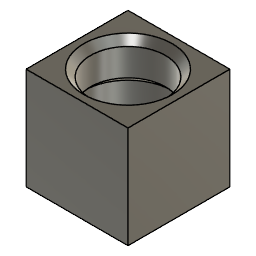
Peg hole_v1 (Autodesk Fusion 360 design; units mm, degrees)
part number: 2026-01-19-15-04-58-543
Autodesk Fusion 360 part; units mm, degrees
sketch "Sketch1" plane through (0, 0, 0) normal (0, 0, 1) x (1, 0, 0)
  line L0 (-19.05, -19.05) -> (19.05, -19.05)
  line L1 (19.05, -19.05) -> (19.05, 19.05)
  line L2 (19.05, 19.05) -> (-19.05, 19.05)
  line L3 (-19.05, 19.05) -> (-19.05, -19.05)
  line L4 (0, 1.75) -> (0, 22.5)
  line L5 (1.75, 0) -> (22.5, 0)
  dimension "d1" = 38.1
  dimension "d2" = 38.1
  constraint horizontal L0
  constraint vertical L1
  constraint horizontal L2
  constraint vertical L3
  constraint symmetric L1 L3 L4
  constraint symmetric L0 L2 L5
  measures "d1" distance of L1 L3
  measures "d2" distance of L0 L2
extrude "Extrude1" add sketch "Sketch1" along normal blind 38.1
sketch "Sketch2" plane through (0, 0, 38.1) normal (0, 0, 1) x (-1, 0, 0)
  line L0 (19.05, -19.05) -> (19.05, 19.05)
  line L1 (19.05, 19.05) -> (-19.05, 19.05)
  line L2 (-19.05, 19.05) -> (-19.05, -19.05)
  line L3 (-19.05, -19.05) -> (19.05, -19.05)
  circle A0 centre (0, 0) radius 13.97
  dimension "d5" = 27.94
  constraint coincident A0.centre origin
  measures "d5" diameter of A0
extrude "Extrude2" cut sketch "Sketch2" against normal blind 25.4 contours A0
sketch "Sketch3" plane through (0, 0, 12.7) normal (0, 0, 1) x (-1, 0, 0)
  circle A0 centre (0, 0) radius 13.97
  circle A1 centre (0, 0) radius 16.51
  dimension "d8" = 2.54
  constraint concentric A0 A1
  measures "d8" distance of A0 A1
extrude "Extrude3" cut sketch "Sketch3" along normal blind 10.16 contours A0 | A1
chamfer "Chamfer1" distance 2.54 angle 45 1 edges at (13.0246, -5.0518, 22.86)
chamfer "Chamfer2" distance 2.54 angle 45 1 edges at (13.0246, -5.0518, 38.1)
